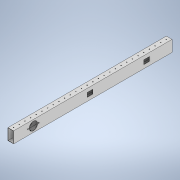
# Autodesk Inventor part: VerseFrame 2021 28in Drive
Saved by Autodesk Inventor 2021 (Build 250183000, 183)
## iProperties
Created: 2020-01-13
Part Number: VerseFrame 2021 28in Drive
Material: Generic
Document SubType Name: Modeling
Designer: aidan
Density: 1 g/cm^3
Appearance: Default
Author: aidan
Autodesk Inventor part; units mm, degrees
ref_plane "YZ Plane" through (0, 0, 0) normal (1, 0, 0) x (0, 1, 0)
ref_plane "XZ Plane" through (0, 0, 0) normal (0, 1, 0) x (-1, 0, 0)
ref_plane "XY Plane" through (0, 0, 0) normal (0, 0, 1) x (1, 0, 0)
sketch "Sketch1" plane through (0, 0, 0) normal (0, 0, 1) x (1, 0, 0)
  line L0 (-12.1708, 16.0073) -> (13.2292, 16.0073)
  line L1 (13.2292, 16.0073) -> (13.2292, -34.7927)
  line L2 (13.2292, -34.7927) -> (-12.1708, -34.7927)
  line L3 (-12.1708, -34.7927) -> (-12.1708, 16.0073)
  line L4 (11.9592, 14.7373) -> (-10.9008, 14.7373)
  line L5 (-10.9008, 14.7373) -> (-10.9008, -33.5227)
  line L6 (-10.9008, -33.5227) -> (11.9592, -33.5227)
  line L7 (11.9592, -33.5227) -> (11.9592, 14.7373)
  point P0 (0, 0)
  dimension "d0" = 25.4
  dimension "d1" = 50.8
  dimension "d2" = 1.27
  constraints: 16 end point, 4 parallel, 2 perpendicular, 1 horizontal, 3 other
  measures "d0" distance of L0.start L0.end
  measures "d1" distance of L0.end L1.end
  measures "d2" distance between parallel lines of L0 L4
extrude "Extrusion1" add sketch "Sketch1" along normal blind 711.2
sketch "Sketch2" plane through (-12.1708, 16.0073, 0) normal (0, 1, 0) x (1, 0, 0)
  circle A0 centre (12.7, -12.7) radius 1.7272
  line L0 (25.4, 0) -> (0, 0) projected
  line L1 (0, 0) -> (0, -711.2) projected
  point P0 (12.1708, 0)
  dimension "d5" = 3.4544
  dimension "d6" = 12.7
  dimension "d7" = 12.7
  constraints: 1 centre point
  measures "d5" diameter of A0
  measures "d6" distance from line of L0 A0.centre
  measures "d7" distance from line of L1 A0.centre
extrude "Extrusion2" cut sketch "Sketch2" against normal through all
pattern_linear "Rectangular Pattern1" count 71 spacing 25.4 along (0, 0, 1) of "Extrusion2"
sketch "Sketch3" plane through (13.2292, -34.7927, 0) normal (1, 0, 0) x (0, 0, -1)
  circle A0 centre (-622.3, 25.4) radius 19.05
  circle A1 centre (-622.3, 25.4) radius 23.8125 construction
  line L0 (-711.2, 1.27) -> (-711.2, 49.53) projected
  line L1 (-711.2, 25.4) -> (0, 25.4) construction
  circle A2 centre (-646.1125, 25.4) radius 2.4892
  circle A3 centre (-598.4875, 25.4) radius 2.4892
  line L2 (-355.6, 34.925) -> (-381, 34.925)
  line L3 (-381, 34.925) -> (-381, 15.875)
  line L4 (-381, 15.875) -> (-355.6, 15.875)
  line L5 (-355.6, 15.875) -> (-355.6, 34.925)
  line L6 (-355.6, 34.925) -> (-381, 15.875) construction
  line L7 (-381, 34.925) -> (-355.6, 15.875) construction
  line L8 (-127, 34.925) -> (-101.6, 34.925)
  line L9 (-101.6, 34.925) -> (-101.6, 15.875)
  line L10 (-101.6, 15.875) -> (-127, 15.875)
  line L11 (-127, 15.875) -> (-127, 34.925)
  line L12 (-127, 34.925) -> (-101.6, 15.875) construction
  line L13 (-101.6, 34.925) -> (-127, 15.875) construction
  circle A4 centre (-622.3, 25.4) radius 76.2 construction
  circle A5 centre (-368.3, 25.4) radius 76.2 construction
  circle A6 centre (-114.3, 25.4) radius 76.2 construction
  point P0 (0, 34.7927)
  dimension "d15" = 47.625
  dimension "d16" = 38.1
  dimension "d17" = 88.9
  dimension "d18" = 4.9784
  dimension "d19" = 152.4
  dimension "d20" = 25.4
  dimension "d21" = 19.05
  dimension "d22" = 254
  dimension "d23" = 254
  constraints: 26 end point, 7 centre point, 5 midpoint, 5 point on line, 4 coincident, 4 parallel, 3 equal radius, 3 horizontal, 2 equal length, 2 perpendicular, 2 point on circle
  measures "d15" diameter of A1
  measures "d16" diameter of A0
  measures "d17" distance from line of L0 A0.centre
  measures "d18" diameter of A3
  measures "d19" diameter of A4
  measures "d20" distance of L2.start L2.end
  measures "d21" distance of L2.end L3.end
  measures "d22" distance of A5.centre A0.centre
  measures "d23" distance of A6.centre point (-368.3, 25.4)
extrude "Extrusion3" cut sketch "Sketch3" against normal blind 25.4
equation "\"d3\" = d13"
equation "\"d10\" = d14"
equation "\"d13\" = 711.2"
equation "\"d14\" = d13"
body "Solid1"
